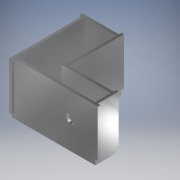
# Autodesk Inventor part: RSX Structure
Saved by Autodesk Inventor 2017 (Build 210142000, 142)
## iProperties
Created: 2016-10-27
Part Number: RSX Structure
Material: Aluminum 6061
Document SubType Name: Modeling
Designer: eschr_000
Density: 2.7 g/cm^3
Appearance: Aluminum - Flat
Mass: 2364.77 g
Surface Area: 2374.75 cm^2
Volume: 875.841 cm^3
Author: eschr_000
Autodesk Inventor part; units mm, degrees
ref_plane "YZ Plane" through (0, 0, 0) normal (1, 0, 0) x (0, 1, 0)
ref_plane "XZ Plane" through (0, 0, 0) normal (0, 1, 0) x (-1, 0, 0)
ref_plane "XY Plane" through (0, 0, 0) normal (0, 0, 1) x (1, 0, 0)
sketch "Sketch2" plane through (0, 0, 0) normal (0, 1, 0) x (-1, 0, 0)
  line L0 (127, 0) -> (177.8, 0)
  line L1 (177.8, 0) -> (177.8, -203.2)
  line L2 (177.8, -203.2) -> (0, -203.2)
  line L3 (0, -203.2) -> (0, -114.3)
  line L4 (0, -114.3) -> (127, -114.3)
  line L5 (127, -114.3) -> (127, 0)
  point P0 (0, 0)
  dimension "d0" = 203.2
  dimension "d1" = 177.8
  dimension "d65" = 50.8
  dimension "d66" = 88.9
  constraints: 12 end point, 2 horizontal, 2 parallel, 2 perpendicular
  measures "d0" distance of L2.end point (0, 0)
  measures "d1" distance of L1.end L2.end
  measures "d65" distance between parallel lines of L1 L5
  measures "d66" distance between parallel lines of L2 L4
extrude "Extrusion1" add sketch "Sketch2" along normal blind 12.7
sketch "Sketch3" plane through (0, 12.7, 0) normal (0, 1, 0) x (1, 0, 0)
  line L0 (-127, 0) -> (-177.8, 0)
  line L1 (-177.8, 0) -> (-177.8, 203.2)
  line L2 (-177.8, 203.2) -> (0, 203.2)
  line L3 (0, 203.2) -> (0, 114.3)
  line L4 (-171.45, 196.85) -> (-171.45, 6.35)
  line L5 (-171.45, 6.35) -> (-133.35, 6.35)
  line L6 (-6.35, 120.65) -> (-6.35, 196.85)
  line L7 (-6.35, 196.85) -> (-171.45, 196.85)
  line L8 (0, 114.3) -> (-127, 114.3)
  line L9 (-127, 114.3) -> (-127, 0)
  line L10 (-6.35, 120.65) -> (-133.35, 120.65)
  line L11 (-133.35, 120.65) -> (-133.35, 6.35)
  line L12 (-127, 0) -> (-127, 114.3) projected
  line L13 (0, 114.3) -> (0, 203.2) projected
  point P0 (0, 0)
  point P1 (-127, 6.35)
  point P2 (0, 120.65)
  point P3 (-114.3, 0)
  point P4 (-6.35, 114.3)
  dimension "d4" = 6.35
  dimension "d61" = 120.65
  dimension "d62" = 107.95
  dimension "d63" = 6.35
  dimension "d64" = 6.35
  dimension "d76" = 0
  dimension "d77" = 6.35
  dimension "d78" = 0
  constraints: 24 end point, 4 parallel, 4 perpendicular, 4 point on line, 3 horizontal
  measures "d4" distance between parallel lines of L1 L4
  measures "d61" distance between parallel lines of L6 L9
  measures "d62" distance between parallel lines of L5 L8
  measures "d63" distance between parallel lines of L8 L10
  measures "d64" distance between parallel lines of L9 L11
  measures "d76" distance between parallel lines of L12 L9
  measures "d77" distance between parallel lines of L3 L6
  measures "d78" distance between parallel lines of L13 L3
extrude "Extrusion2" add sketch "Sketch3" along normal blind 114.3
sketch "Sketch5" plane through (0, 12.7, 0) normal (0, 1, 0) x (1, 0, 0)
  line L0 (-114.3, 114.3) -> (-114.3, 6.35)
  line L1 (-6.35, 120.65) -> (-6.3512, 120.1928)
  line L2 (-171.45, 114.3) -> (-114.3, 114.3)
  line L3 (-171.45, 6.35) -> (-171.45, 196.85) projected
  line L4 (-133.35, 6.35) -> (-171.45, 6.35) projected
  line L5 (-171.45, 120.65) -> (-57.15, 120.65)
  line L6 (-107.95, 114.3) -> (-107.95, 6.35)
  line L7 (-171.45, 120.65) -> (-6.35, 120.65)
  line L8 (-107.95, 114.3) -> (-6.35, 114.3)
  line L9 (-6.35, 196.85) -> (-6.35, 120.65) projected
  line L10 (-171.45, 120.65) -> (-171.45, 114.3)
  line L11 (-6.35, 120.65) -> (-6.35, 114.3)
  line L12 (-6.35, 120.65) -> (-6.35, 114.3)
  line L13 (-133.35, 6.35) -> (-107.95, 6.35)
  line L14 (-171.45, 6.35) -> (-133.35, 6.35) projected
  point P0 (-6.35, 6.35)
  dimension "d37" = 107.95
  dimension "d38" = 6.35
  dimension "d58" = 101.6
  dimension "d60" = 6.35
  constraints: 22 end point, 4 collinear, 2 horizontal, 1 parallel, 1 point on line
  measures "d37" distance between parallel lines of L2 L4
  measures "d38" distance between parallel lines of L2 L5
  measures "d58" distance between parallel lines of L9 L6
  measures "d60" distance between parallel lines of L6 L0
extrude "Extrusion5" [suppressed]
sketch "Sketch6" plane through (0, 0, 0) normal (0, -1, 0) x (1, 0, 0)
  line L0 (0, -203.2) -> (-177.8, 0) construction
  circle A0 centre (-88.9, -101.6) radius 101.6 construction
  line L1 (-177.8, -203.2) -> (0, 0) construction
  point P0 (-155.8041, -178.0618)
  point P1 (-155.8041, -25.1382)
  point P2 (-21.9959, -25.1382)
  point P3 (-21.9959, -178.0618)
  dimension "d25" = 203.2
  constraints: 4 end point, 4 point on circle, 4 point on line, 1 centre point, 1 coincident, 1 midpoint
  measures "d25" diameter of A0
hole "Hole1" [suppressed]
sketch "Sketch7" plane through (-6.35, 12.7, -196.85) normal (-1, 0, 0) x (0, 0, 1)
  line L0 (76.2, 0) -> (0, 0) projected
  line L1 (76.2, 114.3) -> (76.2, 0) projected
  line L2 (0, 0) -> (76.2, 0)
  line L3 (76.2, 0) -> (76.2, 63.5)
  line L4 (76.2, 63.5) -> (0, 63.5)
  line L5 (0, 63.5) -> (0, 0)
  point P0 (196.85, -12.7)
  dimension "d39" = 63.5
  constraints: 8 end point, 2 parallel, 1 horizontal, 1 perpendicular, 1 point on line
  measures "d39" distance of L4.end L0.end
extrude "Extrusion6" [suppressed]
sketch "Sketch10" plane through (0, 12.7, 0) normal (0, 1, 0) x (1, 0, 0)
  line L0 (-164.5, 98.825) -> (-135.392, 98.825) construction
  line L1 (-135.392, 98.825) -> (-135.392, 21.825) construction
  line L2 (-135.392, 21.825) -> (-164.5, 21.825) construction
  line L3 (-164.5, 21.825) -> (-164.5, 98.825) construction
  line L4 (-171.45, 6.35) -> (-171.45, 196.85) projected
  line L5 (-133.35, 114.3) -> (-171.45, 114.3) projected
  line L6 (-171.45, 6.35) -> (-133.35, 6.35) projected
  circle A0 centre (-135.392, 98.825) radius 1.6
  circle A1 centre (-164.5, 98.825) radius 1.6
  circle A2 centre (-135.392, 21.825) radius 1.6
  circle A3 centre (-164.5, 21.825) radius 1.6
  point P0 (0, 0)
  point P1 (-127, 114.3)
  point P2 (-127, 6.35)
  dimension "d40" = 6.95
  dimension "d41" = 29.108
  dimension "d42" = 77
  dimension "d43" = 15.475
  dimension "d44" = 15.475
  dimension "d45" = 3.2
  dimension "d46" = 3.2
  dimension "d47" = 3.2
  dimension "d48" = 3.2
  constraints: 8 end point, 4 centre point, 4 coincident, 2 parallel, 1 horizontal, 1 perpendicular
  measures "d40" distance between parallel lines of L4 L3
  measures "d41" distance of L1.end L2.end
  measures "d42" distance of L2.end L0.start
  measures "d43" distance between parallel lines of L5 L0
  measures "d44" distance between parallel lines of L6 L2
  measures "d45" diameter of A0
  measures "d46" diameter of A1
  measures "d47" diameter of A2
  measures "d48" diameter of A3
extrude "Extrusion7" cut sketch "Sketch10" against normal through all
sketch "Sketch11" plane through (-177.8, 0, -203.2) normal (-1, 0, 0) x (0, 0, 1)
  line L0 (203.2, 0) -> (203.2, 127) projected
  line L1 (203.2, 20.5386) -> (0, 20.5386) construction
  line L2 (0, 0) -> (0, 127) projected
  line L3 (196.85, 127) -> (6.35, 127) projected
  circle A0 centre (142.875, 67.55) radius 10
  line L4 (0, 0) -> (203.2, 0) projected
  point P0 (88.9, 127)
  dimension "d51" = 20
  dimension "d52" = 67.55
  dimension "d53" = 53.975
  dimension "d54" = 53.975
  constraints: 2 end point, 2 point on line, 1 centre point, 1 horizontal
  measures "d51" diameter of A0
  measures "d52" distance from line of L4 A0.centre
  measures "d53" horizontal distance of point (88.9, 127) A0.centre
  measures "d54" horizontal distance of L3.start A0.centre
extrude "Extrusion8" cut sketch "Sketch11" against normal up to surface (6.35 mm away)
sketch "Sketch14" plane through (0, 127, 0) normal (0, 1, 0) x (1, 0, 0)
  line L0 (-177.8, 0) -> (-127, 0) projected
  line L1 (-127, 0) -> (-120.65, 0)
  line L2 (-120.65, 0) -> (-120.65, 6.35)
  line L3 (-120.65, 6.35) -> (-127, 6.35)
  line L4 (-127, 6.35) -> (-127, 0)
  line L5 (-177.8, 0) -> (-171.45, 0)
  line L6 (-171.45, 0) -> (-171.45, -6.35)
  line L7 (-171.45, -6.35) -> (-177.8, -6.35)
  line L8 (-177.8, -6.35) -> (-177.8, 0)
  point P0 (0, 0)
  dimension "d79" = 6.35
  dimension "d80" = 6.35
  dimension "d81" = 6.35
  dimension "d82" = 6.35
  constraints: 16 end point, 4 parallel, 2 horizontal, 2 perpendicular
  measures "d79" distance of L3.end L2.end
  measures "d80" distance between parallel lines of L3 L1
  measures "d81" distance of L6.end L7.end
  measures "d82" distance between parallel lines of L0 L7
extrude "Extrusion11" add sketch "Sketch14" against normal up to surface (114.3 mm away)
sketch "Sketch15" plane through (0, 127, 0) normal (0, 1, 0) x (1, 0, 0)
  circle A0 centre (-135.392, 21.825) radius 1.6 projected
  circle A1 centre (-135.392, 98.825) radius 1.6 projected
  circle A2 centre (-164.5, 98.825) radius 1.6 projected
  circle A3 centre (-164.5, 21.825) radius 1.6 projected
  line L0 (-6.35, 196.85) -> (-171.45, 196.85) projected
  line L1 (-171.45, 196.85) -> (-171.45, 6.35) projected
  line L2 (-171.45, 6.35) -> (-133.35, 6.35) projected
  line L3 (-133.35, 6.35) -> (-133.35, 120.65) projected
  line L4 (-133.35, 120.65) -> (-6.35, 120.65) projected
  line L5 (-6.35, 120.65) -> (-6.35, 196.85) projected
  line L6 (-133.35, 120.65) -> (-127, 120.65)
  line L7 (-127, 120.65) -> (-127, 127)
  line L8 (-127, 127) -> (-133.35, 127)
  line L9 (-133.35, 127) -> (-133.35, 120.65)
  line L10 (-171.45, 196.85) -> (-6.35, 196.85) projected
  line L11 (-6.35, 196.85) -> (-6.35, 120.65) projected
  line L12 (-6.35, 120.65) -> (-133.35, 120.65) projected
  line L13 (-133.35, 120.65) -> (-133.35, 6.35) projected
  line L14 (-133.35, 6.35) -> (-171.45, 6.35) projected
  line L15 (-171.45, 6.35) -> (-171.45, 196.85) projected
  line L16 (-177.8, 203.2) -> (-177.8, -6.35) projected
  line L17 (-177.8, -6.35) -> (-171.45, -6.35) projected
  line L18 (-171.45, -6.35) -> (-171.45, 0) projected
  line L19 (-171.45, 0) -> (-120.65, 0) projected
  line L20 (-120.65, 0) -> (-120.65, 6.35) projected
  line L21 (-120.65, 6.35) -> (-127, 6.35) projected
  line L22 (-127, 6.35) -> (-127, 114.3) projected
  line L23 (-127, 114.3) -> (0, 114.3) projected
  line L24 (0, 114.3) -> (0, 203.2) projected
  line L25 (0, 203.2) -> (-177.8, 203.2) projected
  line L26 (0, 114.3) -> (6.35, 114.3)
  line L27 (6.35, 114.3) -> (6.35, 120.65)
  line L28 (6.35, 120.65) -> (0, 120.65)
  line L29 (0, 120.65) -> (0, 114.3)
  line L30 (0, 114.3) -> (0, 203.2) projected
  line L31 (0, 203.2) -> (-6.35, 203.2)
  line L32 (-6.35, 203.2) -> (-6.35, 209.55)
  line L33 (-6.35, 209.55) -> (0, 209.55)
  line L34 (0, 209.55) -> (0, 203.2)
  line L35 (0, 203.2) -> (-177.8, 203.2) projected
  line L36 (-177.8, 203.2) -> (-184.15, 203.2)
  line L37 (-184.15, 203.2) -> (-184.15, 196.85)
  line L38 (-184.15, 196.85) -> (-177.8, 196.85)
  line L39 (-177.8, 196.85) -> (-177.8, 203.2)
  point P0 (0, 0)
  dimension "d85" = 6.35
  dimension "d86" = 6.35
  dimension "d87" = 6.35
  dimension "d88" = 6.35
  dimension "d89" = 6.35
  dimension "d90" = 6.35
  dimension "d91" = 6.35
  constraints: 32 end point, 8 parallel, 4 horizontal, 4 perpendicular
  measures "d85" distance of L6.end L7.end
  measures "d86" distance between parallel lines of L13 L7
  measures "d87" distance of L28.end L27.end
  measures "d88" distance of L32.end L33.end
  measures "d89" distance of L31.end L32.end
  measures "d90" distance of L38.end L37.end
  measures "d91" distance of L37.end L36.end
extrude "Extrusion12" add sketch "Sketch15" against normal up to surface (114.3 mm away) contours L4 L9 L8 L7 | L16 L38 L37 L36 | L32 L33 L34 L25 | L28 L27 L26 L24
equation "\"d43\" = d44"
equation "\"d53\" = d54"
body "Solid1"
